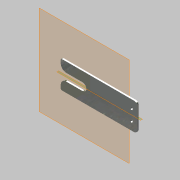
# Autodesk Inventor part: wheel_mount
Saved by Autodesk Inventor 2021.2 (Build 252289000, 289)
## iProperties
Created: 2021-07-08
Part Number: wheel_mount
Material: アルミニウム 6061
Document SubType Name: Modeling
Designer: gisen
Density: 2.7 g/cm^3
Appearance: アルミニウム - フラット
Author: gisen
Autodesk Inventor part; units mm, degrees
ref_plane "YZ Plane" through (0, 0, 0) normal (1, 0, 0) x (0, 1, 0)
ref_plane "XZ Plane" through (0, 0, 0) normal (0, 1, 0) x (-1, 0, 0)
ref_plane "XY Plane" through (0, 0, 0) normal (0, 0, 1) x (1, 0, 0)
ref_plane "作業平面1" through (0, 0, 0) normal (0, 0, 1) x (1, 0, 0)
sketch "スケッチ2" plane through (0, 0, 0) normal (0, 0, 1) x (1, 0, 0)
  line L0 (100, -50) -> (-40, -50)
  line L1 (-40, -50) -> (-40, -100)
  line L2 (-40, -100) -> (100, -100)
  line L3 (100, -100) -> (100, -50)
  circle A0 centre (0, -75) radius 6 construction
  circle A1 centre (0, -75) radius 75 construction
  point P0 (0, 0)
  dimension "d1" = 150
  dimension "d2" = 25
  dimension "d3" = 25
  dimension "d4" = 40
  dimension "d5" = 100
  constraints: 8 end point, 2 parallel, 1 horizontal, 1 perpendicular, 1 vertical alignment
  measures "d2" distance from line of L0 A0.centre
  measures "d3" distance from line of L2 A0.centre
  measures "d4" distance from line of L1 A0.centre
  measures "d5" distance from line of A0.centre L3
extrude "押し出し1" add sketch "スケッチ2" along normal blind 3
sketch "スケッチ3" plane through (0, 0, 3) normal (0, 0, 1) x (1, 0, 0)
  circle A0 centre (0, -75) radius 6 construction
  circle A1 centre (0, -75) radius 7
  line L0 (0, -68) -> (-38.1, -68) construction
  line L1 (-38.1, -68) -> (-38.1, -82) construction
  line L2 (-38.1, -82) -> (0, -82) construction
  line L3 (0, -82) -> (0, -68) construction
  line L4 (0, -68) -> (-40, -68)
  line L5 (-40, -68) -> (-40, -82)
  line L6 (-40, -82) -> (0, -82)
  line L7 (0, -82) -> (0, -68)
  line L8 (-40, -50) -> (-40, -100) projected
  point P0 (0, 0)
  point P1 (0, -82)
  dimension "d8" = 14
  constraints: 16 end point, 4 horizontal, 4 parallel, 2 perpendicular, 1 coincident, 1 collinear, 1 point on line, 3 other
extrude "押し出し2" cut sketch "スケッチ3" against normal blind 14
fillet "フィレット1" radius 10 2 edges at (-40, -68, 1.5) (-40, -82, 1.5)
ref_plane "作業平面2" through (-40, -75, 0) normal (0, -1, 0) x (1, 0, 0)
sketch "スケッチ4" plane through (0, 0, 3) normal (0, 0, 1) x (1, 0, 0)
  arc A0 (88.8653, -83.8021) -> (91.1347, -83.8021) centre (90, -85) ccw construction
  arc A1 (88.8653, -83.8021) -> (91.1347, -83.8021) centre (90, -85) ccw construction
  arc A2 (91.1347, -66.1979) -> (88.8653, -66.1979) centre (90, -65) ccw construction
  point P0 (0, 0)
  constraints: 6 point on circle, 3 centre point, 2 coincident, 10 other
hole "穴1" at (90, -65, 3) at (90, -85, 3) direction (0, 0, -1) diameter 4.5 end through all
fillet "フィレット2" radius 5 2 edges at (100, -50, 1.5) (100, -100, 1.5)
fillet "フィレット2" radius 2 2 edges at (-40, -50, 1.5) (-40, -100, 1.5)
equation "\"d3\" = d2"
equation "\"d9\" = d8"
